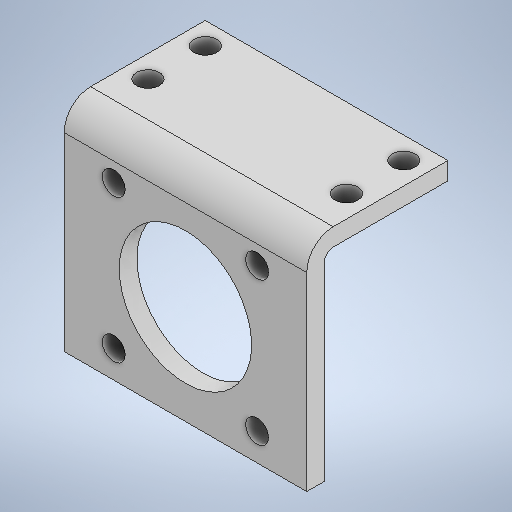
# Autodesk Inventor part: TS_V1_Fallmagazin_Zylinderhalter_int
Saved by Autodesk Inventor 2025.1 (Build 291241000, 241)
## iProperties
Created: 2025-06-13
Part Number: TS_V1_Fallmagazin_Zylinderhalter_int
Material: Generisch
Document SubType Name: Modeling
Designer: tino
Density: 1 g/cm^3
Appearance: Vorgabe
Author: tino
Autodesk Inventor part; units mm, degrees
ref_plane "YZ Plane" through (0, 0, 0) normal (1, 0, 0) x (0, 1, 0)
ref_plane "XZ Plane" through (0, 0, 0) normal (0, 1, 0) x (-1, 0, 0)
ref_plane "XY Plane" through (0, 0, 0) normal (0, 0, 1) x (1, 0, 0)
sketch "Skizze1" plane through (0, 0, 0) normal (1, 0, 0) x (0, 1, 0)
  line L0 (-153.8173, -10.7111) -> (-149.8173, -10.7111)
  line L1 (-149.8173, -10.7111) -> (-149.8173, 38.2889)
  line L2 (-149.8173, 38.2889) -> (-153.8173, 38.2889)
  line L3 (-153.8173, 38.2889) -> (-153.8173, -10.7111)
  line L4 (-153.8173, 38.2889) -> (-121.8173, 38.2889)
  line L5 (-121.8173, 38.2889) -> (-121.8173, 34.2889)
  line L6 (-121.8173, 34.2889) -> (-153.8173, 34.2889)
  line L7 (-153.8173, 34.2889) -> (-153.8173, 38.2889)
  point P0 (0, 0)
  point P1 (-149.8173, 34.2889)
  point P2 (-151.8173, -10.7111)
  dimension "d0" = 4
  dimension "d2" = 32
  dimension "d3" = 4
  dimension "d10" = 45
  constraints: 16 end point, 4 parallel, 2 horizontal, 2 perpendicular, 1 midpoint
  measures "d0" distance of L2.end L1.end
  measures "d2" distance of L5.end L6.end
  measures "d3" distance of L4.end L5.end
  measures "d10" distance from line of point (-151.817, -10.711) L6
extrude "Extrusion1" add sketch "Skizze1" along normal blind 55
fillet "Rundung1" radius 2 1 edges at (27.5, -149.8173, 34.2889)
fillet "Rundung2" radius 6 1 edges at (27.5, -153.8173, 38.2889)
sketch "Skizze2" plane through (0, -149.8173, -10.7111) normal (0, 1, 0) x (1, 0, 0)
  line L0 (0, -45) -> (55, -45) projected
  line L1 (55, -43) -> (0, -43) projected
  line L2 (55, 0) -> (55, -43) projected
  point P0 (0, -10.7111)
  point P1 (43.75, -38.75)
  dimension "d9" = 4.25
  dimension "d24" = 11.25
  measures "d9" distance from line of L1 point (43.75, -38.75)
  measures "d24" distance from line of L2 point (43.75, -38.75)
hole "Bohrung1" at (43.75, -149.8173, 28.0389) direction (0, -1, 0) diameter 5.2 end through all
pattern_linear "Rechteckige Anordnung1" count 2 spacing 32.5 along (-1, 0, 0) count 2 spacing 32.5 along (0, 0, -1) of "Bohrung1"
sketch "Skizze3" plane through (55, -121.8173, 34.2889) normal (0, 0, -1) x (-1, 0, 0)
  line L0 (55, -28) -> (0, -28) projected
  line L1 (55, -26) -> (0, -26) projected
  line L2 (0, -26) -> (0, 0) projected
  point P0 (55, 121.8173)
  point P1 (5, -18)
  dimension "d27" = 5
  dimension "d28" = 10
  measures "d27" distance from line of L2 point (5, -18)
  measures "d28" distance from line of point (5, -18) L0
hole "Bohrung2" at (50, -139.8173, 34.2889) direction (0, 0, 1) diameter 5.2 end through all
pattern_linear "Rechteckige Anordnung2" count 2 spacing 13 along (0, 1, 0) count 2 spacing 45 along (-1, 0, 0) of "Bohrung2"
sketch "Skizze4" plane through (0, -149.8173, -10.7111) normal (0, 1, 0) x (1, 0, 0)
  circle A0 centre (43.75, -38.75) radius 2.6 construction
  circle A1 centre (11.25, -6.25) radius 2.6 construction
  line L0 (43.75, -38.75) -> (11.25, -38.75) construction
  line L1 (11.25, -38.75) -> (11.25, -6.25) construction
  line L2 (11.25, -6.25) -> (43.75, -6.25) construction
  line L3 (43.75, -6.25) -> (43.75, -38.75) construction
  line L4 (43.75, -38.75) -> (11.25, -6.25) construction
  line L5 (43.75, -6.25) -> (11.25, -38.75) construction
  circle A2 centre (27.5, -22.5) radius 15
  point P0 (0, -10.7111)
  dimension "d42" = 30
  constraints: 12 end point, 2 parallel, 2 perpendicular, 1 centre point, 1 horizontal, 1 midpoint
  measures "d42" diameter of A2
extrude "Extrusion2" cut sketch "Skizze4" against normal through all
